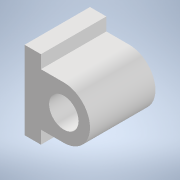
# Autodesk Inventor part: PillowBlock
Saved by Autodesk Inventor 2020 (Build 240168000, 168)
## iProperties
Created: 2020-03-07
Part Number: PillowBlock
Material: Nylon, molybdenum disulphide
Document SubType Name: Modeling
Designer: 10300812
Mass: 11.6248 g
Surface Area: 43.2804 cm^2
Volume: 10.2874 cm^3
Density: 1.13 g/cm^3
Appearance: Nylon 6
Author: 10300812
Autodesk Inventor part; units mm, degrees
ref_plane "YZ Plane" through (0, 0, 0) normal (1, 0, 0) x (0, 1, 0)
ref_plane "XZ Plane" through (0, 0, 0) normal (0, 1, 0) x (-1, 0, 0)
ref_plane "XY Plane" through (0, 0, 0) normal (0, 0, 1) x (1, 0, 0)
sketch "Sketch1" plane through (0, 0, 0) normal (0, 0, 1) x (1, 0, 0)
  circle A0 centre (0, 0) radius 4.5
  arc A1 (0, -8) -> (0, 8) centre (0, 0) ccw
  line L0 (0, 8) -> (-9, 8)
  line L1 (-9, 8) -> (-9, 13.5)
  line L2 (-9, 13.5) -> (-15, 13.5)
  line L3 (-15, 13.5) -> (-15, -13.5)
  line L4 (-15, -13.5) -> (-9, -13.5)
  line L5 (-9, -13.5) -> (-9, -8)
  line L6 (-9, -8) -> (0, -8)
  dimension "d0" = 9
  dimension "d1" = 16
  dimension "d2" = 6
  dimension "d3" = 15
  dimension "d6" = 27
  constraints: 14 end point, 4 perpendicular, 2 centre point, 2 coincident, 2 point on circle, 2 point on line, 2 vertical alignment, 1 collinear, 1 horizontal, 1 tangent
  measures "d0" diameter of A0
  measures "d1" diameter of A1
  measures "d2" distance of L1.end L2.end
  measures "d3" distance from line of point (0, 0) L3
  measures "d6" distance of L2.end L3.end
extrude "Extrusion1" add sketch "Sketch1" along normal mid plane 30
body "Solid1"
